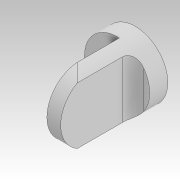
# Autodesk Inventor part: Link3
Saved by Autodesk Inventor 2020 (Build 240168000, 168)
## iProperties
Created: 2021-03-25
Part Number: Link3
Material: Generic
Document SubType Name: Modeling
Designer: DDeGo
Density: 1 g/cm^3
Appearance: Default
Author: DDeGo
Autodesk Inventor part; units mm, degrees
ref_plane "YZ Plane" through (0, 0, 0) normal (1, 0, 0) x (0, 1, 0)
ref_plane "XZ Plane" through (0, 0, 0) normal (0, 1, 0) x (-1, 0, 0)
ref_plane "XY Plane" through (0, 0, 0) normal (0, 0, 1) x (1, 0, 0)
sketch "Sketch1" plane through (0, 0, 0) normal (1, 0, 0) x (0, 1, 0)
  circle A0 centre (0, 0) radius 25
  arc A1 (45, 0) -> (-45, 0) centre (0, 0) ccw
  line L0 (45, 0) -> (-45, 0) construction
  line L1 (-45, 0) -> (-45, -55)
  line L2 (-45, -55) -> (45, -55)
  line L3 (45, -55) -> (45, 0)
  dimension "d0" = 50
  dimension "d1" = 90
  dimension "d4" = 55
  constraints: 8 end point, 2 centre point, 2 coincident, 2 parallel, 2 point on circle, 1 horizontal, 1 midpoint, 1 perpendicular
  measures "d0" diameter of A0
  measures "d1" diameter of A1
  measures "d4" distance from line of L2 point (0, 0)
extrude "Extrusion1" add sketch "Sketch1" along normal mid plane 19
sketch "Sketch2" plane through (-9.5, -45, -55) normal (0, 0, -1) x (-1, 0, 0)
  line L0 (-9.5, 45) -> (3, 45) construction
  circle A0 centre (3, 45) radius 45
  dimension "d5" = 90
  dimension "d9" = 12.5
  constraints: 2 end point, 1 centre point, 1 coincident, 1 horizontal
  measures "d5" diameter of A0
  measures "d9" distance of L0.start L0.end
extrude "Extrusion2" add sketch "Sketch2" along normal blind 25
sketch "Sketch3" plane through (-12.5, 0, -80) normal (0, 0, -1) x (-1, 0, 0)
  line L0 (-21, -21) -> (21, -21)
  line L1 (21, -21) -> (21, 21)
  line L2 (21, 21) -> (-21, 21)
  line L3 (-21, 21) -> (-21, -21)
  circle A0 centre (0, 0) radius 45 projected
  line L4 (-21, -21) -> (21, 21) construction
  line L5 (21, -21) -> (-21, 21) construction
  point P0 (-12.5, 0)
  dimension "d10" = 42
  constraints: 12 end point, 2 midpoint, 2 parallel, 2 perpendicular, 1 horizontal
  measures "d10" distance of L1.end L2.end
extrude "Extrusion3" cut sketch "Sketch3" against normal blind 22 contours L3 L2 L1 L0
sketch "Sketch4" plane through (-12.5, 0, -80) normal (0, 0, -1) x (-1, 0, 0)
  circle A0 centre (0, 0) radius 45 projected
  circle A1 centre (0, 0) radius 29.5
  circle A2 centre (0, 0) radius 43
  point P0 (-12.5, 0)
  dimension "d15" = 86
  dimension "d16" = 59
  constraints: 2 centre point, 2 coincident
  measures "d15" diameter of A2
  measures "d16" diameter of A1
extrude "Extrusion4" cut sketch "Sketch4" against normal blind 4 contours A2
sketch "Sketch5" plane through (9.5, -45, -55) normal (0, 0, -1) x (-1, 0, 0)
  arc A0 (19, 89.899889) -> (0, 84.255573) centre (22, 45) ccw
  line L0 (0, 0) -> (0, 5.744427)
  arc A1 (19, 89.899889) -> (0, 84.255573) centre (22, 45) ccw
  line L1 (0, 84.255573) -> (0, 90)
  arc A2 (0, 5.744427) -> (19, 0.100111) centre (22, 45) ccw
  line L2 (0, 0) -> (0, 5.744427)
  line L3 (19, 0) -> (0, 0)
  line L4 (0, 90) -> (19, 90)
  arc A3 (0, 5.744427) -> (19, 0.100111) centre (22, 45) ccw
  line L5 (0, 90) -> (19, 90)
  line L6 (0, 84.255573) -> (0, 90)
  line L7 (19, 0) -> (0, 0)
  line L8 (19, 90) -> (19, 89.899889)
  line L9 (19, 0.100111) -> (19, 0)
  line L10 (19, 90) -> (19, 89.899889)
  line L11 (19, 0.100111) -> (19, 0)
extrude "Extrusion5" cut sketch "Sketch5" against normal through all
fillet "Fillet2" radius 15 1 edges at (9.5, 0, -55)
sketch "Sketch6" plane through (9.5, 0, 0) normal (1, 0, 0) x (0, 0, -1)
  circle A0 centre (0, 0) radius 25 projected
extrude "Extrusion6" add sketch "Sketch6" against normal up to surface (19 mm away)
sketch "Sketch7" plane through (-9.5, 0, 0) normal (-1, 0, 0) x (0, 0, 1)
  circle A0 centre (0, 0) radius 17.45
  dimension "d24" = 34.9
  constraints: 1 centre point, 1 coincident
  measures "d24" diameter of A0
extrude "Extrusion7" add sketch "Sketch7" along normal blind 7
sketch "Sketch8" plane through (-16.5, 0, 0) normal (-1, 0, 0) x (0, 0, 1)
  line L0 (0, 0) -> (13, 0) construction
  circle A0 centre (13, 0) radius 2.55
  circle A1 centre (6.5, 11.25833) radius 2.55
  circle A2 centre (-6.5, 11.25833) radius 2.55
  circle A3 centre (-13, 0) radius 2.55
  circle A4 centre (-6.5, -11.25833) radius 2.55
  circle A5 centre (6.5, -11.25833) radius 2.55
  dimension "d27" = 5.1
  dimension "d28" = 13
  dimension "d31" = 360
  constraints: 6 centre point, 2 end point, 1 coincident, 1 horizontal, 13 other
  measures "d27" diameter of A0
  measures "d28" distance of L0.start L0.end
extrude "Extrusion8" cut sketch "Sketch8" against normal blind 7.5
ref_plane "Work Plane1" through (0.5, 0, 0) normal (-1, 0, 0) x (0, 0, 1)
sketch "Sketch9" plane through (0.5, 0, 0) normal (-1, 0, 0) x (0, 0, 1)
  circle A0 centre (0, 0) radius 17.45
  line L0 (0, 0) -> (-125.538657, 0) construction
  line L1 (0, 7.5) -> (-125.538657, 7.5)
  line L2 (-125.538657, -7.5) -> (0, -7.5)
  arc A1 (0, -7.5) -> (0, 7.5) centre (0, 0) ccw
  arc A2 (-125.538657, 7.5) -> (-125.538657, -7.5) centre (-125.538657, 0) ccw
  point P0 (-62.769328, 0)
  point P1 (-15.756031, -7.5)
  point P2 (-15.756031, 7.5)
  dimension "d36" = 7.5
  constraints: 8 end point, 4 point on circle, 4 tangent, 2 centre point, 1 horizontal, 1 midpoint, 1 parallel
  measures "d36" radius of A2
extrude "Extrusion9" cut sketch "Sketch9" along normal mid plane 7.5 contours L1 A1 L2 A0 | A0 L2 A2 L1 picked at (-5.816667, 0)
sketch "Sketch10" plane through (-16.5, 0, 0) normal (-1, 0, 0) x (0, 0, 1)
  arc A0 (0, -7.5) -> (0, 7.5) centre (0, 0) ccw projected
  circle A1 centre (0, 0) radius 7.5
  constraints: 1 coincident, 3 other
extrude "Extrusion10" cut sketch "Sketch10" against normal up to surface (20.75 mm away)
sketch "Sketch11" plane through (-12.5, 0, -58) normal (0, 0, -1) x (-1, 0, 0)
  line L0 (-16.75, -7.5) -> (-9.25, -7.5) projected
  line L1 (21, -21) -> (-21, -21) projected
  line L2 (-16.75, -7.5) -> (-9.25, -7.5)
  line L3 (-9.25, -7.5) -> (-9.25, -21)
  line L4 (-9.25, -21) -> (-16.75, -21)
  line L5 (-16.75, -21) -> (-16.75, -7.5)
  point P0 (-12.5, 0)
  constraints: 8 end point, 2 parallel, 1 horizontal, 1 perpendicular, 1 point on line
extrude "Extrusion11" cut sketch "Sketch11" against normal blind 7.5
sketch "Sketch12" plane through (-9.5, -45, -80) normal (0, 0, -1) x (-1, 0, 0)
  arc A0 (-17.718349, 24) -> (23.718349, 24) centre (3, 45) ccw
  line L0 (-13.75, 24) -> (-13.75, 20.716518)
  arc A1 (-17.718349, 24) -> (23.718349, 24) centre (3, 45) ccw
  line L1 (-13.75, 24) -> (-6.25, 24)
  line L2 (-6.25, 24) -> (-6.25, 16.987726)
  point P0 (-9.5, 45)
  point P1 (-13.75, 20.716518)
  constraints: 6 end point, 2 point on circle, 1 horizontal, 1 perpendicular, 1 vertical
extrude "Extrusion12" cut sketch "Sketch12" against normal up to surface (29.5 mm away)
fillet "Fillet3" radius 5 6 edges at (0.5, -7.5, -50.5) (0.633, -26.4154, -50.5) (-3.25, 0, -7.5) (4.25, -7.5, -25.25) (4.25, 7.5, -29) (4.25, 0, 7.5)
fillet "Fillet4" radius 2 1 edges at (-9.5, 0, -17.45)
chamfer "Chamfer1" distance 15 angle 45 1 edges at (-3.25, -24.5061, -80)
sketch "Sketch13" plane through (-9.5, -45, -80) normal (0, 0, -1) x (-1, 0, 0)
  line L0 (-13.75, 20.716518) -> (-13.75, 24)
  line L1 (-13.75, 24) -> (-17.718349, 24)
  arc A0 (-17.718349, 24) -> (-13.75, 20.716518) centre (3, 45) ccw
  point P0 (-9.5, 45)
extrude "Extrusion13" cut sketch "Sketch13" against normal up to surface (4 mm away)
body "Solid1"
